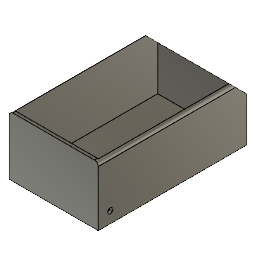
auto v2 (Autodesk Fusion 360 design; units mm, degrees)
Autodesk Fusion 360 part; units mm, degrees
box "BoxPrimitive1" add length 200 width 120 height 80 placed x (0, 1, 0) y (-1, 0, 0) z (0, 0, 1) at (20, 0, 0)
form "Form1" [no effect]
shell "Shell1" thickness 4 removed faces 1 at (-60, 66.6667, 80)
hole "Hole1" at (-100, 16.5108, 15.8612) direction (1, 0, 0) diameter 7 depth 45 tip angle 118
hole "Hole2" at (20, 16.1148, 15.4106) direction (-1, 0, 0) diameter 7 depth 45 tip angle 118
chamfer "Chamfer1" distance 20 angle 45 1 edges at (-40, 200, 80)
fillet "Fillet1" radius 5 1 edges at (-100, 90, 80)
fillet "Fillet2" radius 5 1 edges at (20, 90, 80)
